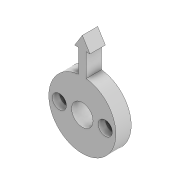
# Autodesk Inventor part: Brushless_Motor_Base_Arrow
Saved by Autodesk Inventor 2020 (Build 240168000, 168)
## iProperties
Created: 2020-05-25
Part Number: Brushless_Motor_Base_Arrow
Material: Generic
Document SubType Name: Modeling
Designer: Shay
Density: 1 g/cm^3
Appearance: Default
Author: Shay
Autodesk Inventor part; units mm, degrees
ref_plane "YZ Plane" through (0, 0, 0) normal (1, 0, 0) x (0, 1, 0)
ref_plane "XZ Plane" through (0, 0, 0) normal (0, 1, 0) x (-1, 0, 0)
ref_plane "XY Plane" through (0, 0, 0) normal (0, 0, 1) x (1, 0, 0)
sketch "Sketch1" plane through (0, 0, 0) normal (0, 0, 1) x (1, 0, 0)
  circle A0 centre (0, 0) radius 13.8811
  circle A1 centre (0, 0) radius 4.445
  circle A2 centre (-9.4996, 0) radius 1.7018
  circle A3 centre (9.4996, 0) radius 1.7018
  dimension "d0" = 27.7622
  dimension "d1" = 8.89
  dimension "d2" = 18.9992
  dimension "d3" = 9.4996
  dimension "d4" = 3.4036
  dimension "d5" = 3.4036
  constraints: 4 centre point, 2 coincident, 2 horizontal alignment
  measures "d0" diameter of A0
  measures "d1" diameter of A1
  measures "d2" distance of A3.centre A2.centre
  measures "d3" distance of point (0, 0) A2.centre
  measures "d4" diameter of A2
  measures "d5" diameter of A3
extrude "Extrusion1" add sketch "Sketch1" along normal blind 6.35
sketch "Sketch2" plane through (0, 0, 6.35) normal (0, 0, 1) x (1, 0, 0)
  line L0 (-1.5875, 4.445) -> (1.5875, 4.445)
  line L1 (1.5875, 4.445) -> (1.5875, 23.4061)
  line L2 (1.5875, 23.4061) -> (-1.5875, 23.4061)
  line L3 (-1.5875, 23.4061) -> (-1.5875, 4.445)
  circle A0 centre (0, 0) radius 4.445 projected
  circle A1 centre (0, 0) radius 13.8811 projected
  line L4 (0, 23.4061) -> (-3.175, 23.4061)
  line L5 (-3.175, 23.4061) -> (0, 28.4861)
  line L6 (0, 23.4061) -> (0, 21.3049) construction
  line L7 (0, 23.4061) -> (3.175, 23.4061)
  line L8 (3.175, 23.4061) -> (0, 28.4861)
  point P0 (0, 4.445)
  dimension "d8" = 3.175
  dimension "d9" = 9.525
  dimension "d10" = 5.08
  dimension "d11" = 3.175
  constraints: 18 end point, 3 parallel, 2 midpoint, 1 horizontal, 1 perpendicular, 1 point on line, 1 symmetric about line, 1 tangent, 1 vertical alignment
  measures "d8" distance of L0.start L0.end
  measures "d9" distance edge to line of A1 L2
  measures "d10" distance from line of L2 L5.end
  measures "d11" distance of L4.start L4.end
extrude "Extrusion2" add sketch "Sketch2" against normal up to surface (6.35 mm away) contours L3 A1 L1 L0 | L3 L2 L1 A1 | L4 L5 L8 L7 L2 picked at (-1.0583, 7.56)
sketch "Sketch3" plane through (0, 0, 6.35) normal (0, 0, 1) x (1, 0, 0)
  circle A0 centre (-9.4996, 0) radius 1.7018 projected
  circle A1 centre (-9.4996, 0) radius 2.921
  circle A2 centre (9.4996, 0) radius 1.7018 projected
  circle A3 centre (9.4996, 0) radius 2.921
  point P0 (0, 0)
  dimension "d14" = 5.842
  dimension "d15" = 5.842
  constraints: 2 centre point, 2 coincident
  measures "d14" diameter of A1
  measures "d15" diameter of A3
extrude "Extrusion3" cut sketch "Sketch3" against normal blind 3.048
equation "\"d3\" = 0.5 * d2"
equation "\"d15\" = d14"
body "Solid1"
